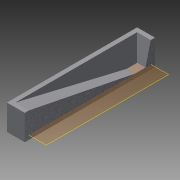
# Autodesk Inventor part: Mould Design 2
Saved by Autodesk Inventor 2015 SP1 (Build 190203100, 203)
## iProperties
Created: 2015-01-22
Part Number: Mould Design 2
Material: Generic
Document SubType Name: Modeling
Designer: I Rabey
Density: 1 g/cm^3
Appearance: Default
Author: I Rabey
Autodesk Inventor part; units mm, degrees
ref_plane "YZ Plane" through (0, 0, 0) normal (1, 0, 0) x (0, 1, 0)
ref_plane "XY Plane" through (0, 0, 0) normal (0, 0, 1) x (1, 0, 0)
sketch "Sketch1" plane through (0, 0, 0) normal (0, 1, 0) x (-1, 0, 0)
  line L0 (-17, 61.5) -> (17, 61.5)
  line L1 (17, 61.5) -> (17, -61.5)
  line L2 (17, -61.5) -> (-17, -61.5)
  line L3 (-17, -61.5) -> (-17, 61.5)
  line L4 (-17, 61.5) -> (17, -61.5) construction
  line L5 (17, 61.5) -> (-17, -61.5) construction
  point P0 (0, 0)
  dimension "d0" = 34
  dimension "d1" = 123
  constraints: 12 end point, 2 midpoint, 2 parallel, 1 horizontal, 1 perpendicular
  measures "d0" distance of L1.end L2.end
  measures "d1" distance of L0.end L1.end
extrude "Extrusion1" add sketch "Sketch1" along normal blind 24
ref_plane "Work Plane1" through (0, 4, 0) normal (0, 1, 0) x (-1, 0, 0)
sketch "Sketch2" plane through (0, 4, 0) normal (0, 1, 0) x (-1, 0, 0)
  line L0 (8, -52.5) -> (-8, -52.5)
  line L1 (-8, -52.5) -> (-8, -42.5)
  line L2 (-8, -42.5) -> (8, -42.5)
  line L3 (8, -42.5) -> (8, -52.5)
  line L4 (-17, -61.5) -> (17, -61.5) projected
  line L5 (17, 61.5) -> (17, -61.5) projected
  point P0 (0, 0)
  dimension "d5" = 16
  dimension "d6" = 10
  dimension "d7" = 9
  dimension "d16" = 9
  constraints: 8 end point, 2 parallel, 1 horizontal, 1 perpendicular
  measures "d5" distance of L1.end L2.end
  measures "d6" distance of L0.end L1.end
  measures "d7" distance between parallel lines of L4 L0
  measures "d16" distance between parallel lines of L5 L3
sketch "Sketch3" plane through (0, 24, 0) normal (0, 1, 0) x (1, 0, 0)
  line L0 (-13, -57.5) -> (13, -57.5)
  line L1 (13, -57.5) -> (13, 57.5)
  line L2 (13, 57.5) -> (-13, 57.5)
  line L3 (-13, 57.5) -> (-13, -57.5)
  line L4 (-17, 61.5) -> (17, 61.5) projected
  line L5 (17, 61.5) -> (17, -61.5) projected
  line L6 (-17, -61.5) -> (17, -61.5) projected
  point P0 (0, 0)
  dimension "d8" = 4
  dimension "d9" = 115
  dimension "d10" = 26
  dimension "d11" = 4
  dimension "d17" = 4
  constraints: 8 end point, 2 parallel, 1 horizontal, 1 perpendicular
  measures "d8" distance between parallel lines of L4 L2
  measures "d9" distance of L0.end L1.end
  measures "d10" distance of L0.start L0.end
  measures "d11" distance between parallel lines of L5 L1
  measures "d17" distance between parallel lines of L6 L0
loft "Loft1" cut profiles "Sketch2", "Sketch3"
body "Solid1"
